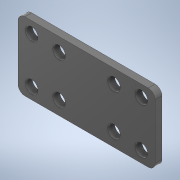
# Autodesk Inventor part: De lot vitme
Saved by Autodesk Inventor 2020 (Build 240168000, 168)
## iProperties
Created: 2021-05-31
Part Number: De lot vitme
Material: Generic
Document SubType Name: Modeling
Designer: Admin
Density: 1 g/cm^3
Appearance: Smooth - Black
Author: Admin
Autodesk Inventor part; units mm, degrees
ref_plane "YZ Plane" through (0, 0, 0) normal (1, 0, 0) x (0, 1, 0)
ref_plane "XZ Plane" through (0, 0, 0) normal (0, 1, 0) x (-1, 0, 0)
ref_plane "XY Plane" through (0, 0, 0) normal (0, 0, 1) x (1, 0, 0)
sketch "Sketch1" plane through (0, 0, 0) normal (0, 0, 1) x (1, 0, 0)
  line L0 (-30, -15) -> (30, -15)
  line L1 (30, -15) -> (30, 15)
  line L2 (30, 15) -> (-30, 15)
  line L3 (-30, 15) -> (-30, -15)
  line L4 (-30, -15) -> (30, 15) construction
  line L5 (30, -15) -> (-30, 15) construction
  line L6 (-12, -9) -> (12, -9)
  line L7 (12, -9) -> (12, 9)
  line L8 (12, 9) -> (-12, 9)
  line L9 (-12, 9) -> (-12, -9)
  line L10 (-12, -9) -> (12, 9) construction
  line L11 (12, -9) -> (-12, 9) construction
  circle A0 centre (-12, 9) radius 2.75
  circle A1 centre (12, 9) radius 2.75
  circle A2 centre (-12, -9) radius 2.75
  circle A3 centre (12, -9) radius 2.75
  point P0 (0, 0)
  dimension "d0" = 60
  dimension "d1" = 30
  dimension "d2" = 24
  dimension "d3" = 18
  dimension "d4" = 5.5
  dimension "d5" = 5.5
  dimension "d6" = 5.5
  dimension "d7" = 5.5
  constraints: 24 end point, 4 centre point, 4 midpoint, 4 parallel, 3 coincident, 2 horizontal, 2 perpendicular
  measures "d0" distance of L2.end L1.end
  measures "d1" distance of L1.end L0.end
  measures "d2" distance of L8.end L7.end
  measures "d3" distance of L7.end L6.end
  measures "d4" diameter of A0
  measures "d5" diameter of A1
  measures "d6" diameter of A2
  measures "d7" diameter of A3
extrude "Extrusion1" add sketch "Sketch1" along normal blind 3 contours L3 L2 L1 L0 | A2 L9 A0 L8 A1 L7 A3 L6
sketch "Sketch2" plane through (0, 0, 3) normal (0, 0, 1) x (1, 0, 0)
  circle A0 centre (-24, 10) radius 2.75
  circle A1 centre (-24, -10) radius 2.75
  line L0 (-30, 15) -> (-30, -15) projected
  circle A2 centre (24, 10) radius 2.75
  circle A3 centre (24, -10) radius 2.75
  line L1 (30, -15) -> (30, 15) projected
  point P0 (0, 0)
  dimension "d10" = 5.5
  dimension "d11" = 5.5
  dimension "d12" = 10
  dimension "d13" = 6
  dimension "d14" = 6
  dimension "d15" = 10
  dimension "d16" = 5.5
  dimension "d17" = 5.5
  dimension "d18" = 20
  dimension "d19" = 10
  dimension "d20" = 6
  dimension "d21" = 6
  constraints: 4 centre point
  measures "d10" diameter of A0
  measures "d11" diameter of A1
  measures "d12" vertical distance of A0.centre point (0, 0)
  measures "d13" distance from line of L0 A0.centre
  measures "d14" distance from line of L0 A1.centre
  measures "d15" vertical distance of point (0, 0) A1.centre
  measures "d16" diameter of A2
  measures "d17" diameter of A3
  measures "d18" distance of A3.centre A2.centre
  measures "d19" vertical distance of point (0, 0) A2.centre
  measures "d20" distance from line of A2.centre L1
  measures "d21" distance from line of L1 A3.centre
extrude "Extrusion2" cut sketch "Sketch2" against normal blind 3
fillet "Fillet1" radius 3 4 edges at (30, 15, 1.5) (30, -15, 1.5) (-30, -15, 1.5) (-30, 15, 1.5)
body "Solid1"
